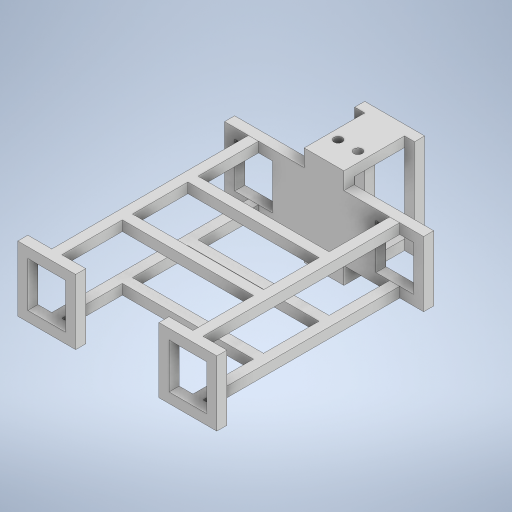
# Autodesk Inventor part: MTail
Saved by Autodesk Inventor 2024 (Build 280153000, 153)
## iProperties
Created: 2023-06-14
Part Number: MTail
Material: Generic
Document SubType Name: Modeling
Designer: vilas
Density: 1 g/cm^3
Appearance: Default
Author: vilas
Autodesk Inventor part; units mm, degrees
sketch "Sketch1" plane through (0, 0, 0) normal (0, 0, 1) x (1, 0, 0)
  line L0 (-32.5, 11.15) -> (32.5, 11.15) construction
  line L1 (32.5, 11.15) -> (32.5, -11.15) construction
  line L2 (32.5, -11.15) -> (-32.5, -11.15) construction
  line L3 (-32.5, -11.15) -> (-32.5, 11.15) construction
  line L4 (-32.5, 11.15) -> (32.5, -11.15) construction
  line L5 (32.5, 11.15) -> (-32.5, -11.15) construction
  line L6 (-32.5, 11.15) -> (-37.5, 11.15)
  line L7 (-37.5, 11.15) -> (-37.5, 16.15)
  line L8 (-37.5, 16.15) -> (-32.5, 16.15)
  line L9 (-32.5, 16.15) -> (-32.5, 11.15)
  line L10 (32.5, 11.15) -> (37.5, 11.15)
  line L11 (37.5, 11.15) -> (37.5, 16.15)
  line L12 (37.5, 16.15) -> (32.5, 16.15)
  line L13 (32.5, 16.15) -> (32.5, 11.15)
  line L14 (32.5, -11.15) -> (37.5, -11.15)
  line L15 (37.5, -11.15) -> (37.5, -16.15)
  line L16 (37.5, -16.15) -> (32.5, -16.15)
  line L17 (32.5, -16.15) -> (32.5, -11.15)
  line L18 (-32.5, -11.15) -> (-37.5, -11.15)
  line L19 (-37.5, -11.15) -> (-37.5, -16.15)
  line L20 (-37.5, -16.15) -> (-32.5, -16.15)
  line L21 (-32.5, -16.15) -> (-32.5, -11.15)
  point P0 (0, 0)
  dimension "d0" = 65
  dimension "d1" = 22.3
  dimension "d2" = 5
  dimension "d3" = 5
  dimension "d4" = 5
  dimension "d5" = 5
  dimension "d6" = 5
  dimension "d7" = 5
  dimension "d8" = 5
  dimension "d9" = 5
  constraints: 44 end point, 10 parallel, 5 horizontal, 5 perpendicular, 2 midpoint
  measures "d0" distance of L1.end L2.end
  measures "d1" distance of L0.end L1.end
  measures "d2" distance of L7.end L8.end
  measures "d3" distance of L6.end L7.end
  measures "d4" distance of L12.end L11.end
  measures "d5" distance of L11.end L10.end
  measures "d6" distance of L15.end L16.end
  measures "d7" distance of L14.end L15.end
  measures "d8" distance of L20.end L19.end
  measures "d9" distance of L19.end L18.end
extrude "Extrusion1" add sketch "Sketch1" along normal mid plane 97.524
ref_plane "Work Plane1" through (0, 0, 48.762) normal (0, 0, 1) x (1, 0, 0)
sketch "Sketch2" plane through (0, 0, 48.762) normal (0, 0, 1) x (1, 0, 0)
  line L0 (0, 0) -> (-35, 0) construction
  line L1 (0, 0) -> (35, 0) construction
  line L2 (-49.35, 16.15) -> (-20.65, 16.15)
  line L3 (-20.65, 16.15) -> (-20.65, -16.15)
  line L4 (-20.65, -16.15) -> (-49.35, -16.15)
  line L5 (-49.35, -16.15) -> (-49.35, 16.15)
  line L6 (-49.35, 16.15) -> (-20.65, -16.15) construction
  line L7 (-20.65, 16.15) -> (-49.35, -16.15) construction
  line L8 (20.65, 16.15) -> (49.35, 16.15)
  line L9 (49.35, 16.15) -> (49.35, -16.15)
  line L10 (49.35, -16.15) -> (20.65, -16.15)
  line L11 (20.65, -16.15) -> (20.65, 16.15)
  line L12 (20.65, 16.15) -> (49.35, -16.15) construction
  line L13 (49.35, 16.15) -> (20.65, -16.15) construction
  line L14 (-25.65, 11.15) -> (-44.35, 11.15)
  line L15 (-44.35, 11.15) -> (-44.35, -11.15)
  line L16 (-44.35, -11.15) -> (-25.65, -11.15)
  line L17 (-25.65, -11.15) -> (-25.65, 11.15)
  line L18 (44.35, 11.15) -> (25.65, 11.15)
  line L19 (25.65, 11.15) -> (25.65, -11.15)
  line L20 (25.65, -11.15) -> (44.35, -11.15)
  line L21 (44.35, -11.15) -> (44.35, 11.15)
  dimension "d13" = 35
  dimension "d14" = 35
  dimension "d15" = 28.7
  dimension "d16" = 32.3
  dimension "d17" = 28.7
  dimension "d18" = 32.3
  dimension "d19" = 5
  dimension "d20" = 5
  constraints: 44 end point, 8 parallel, 4 horizontal, 4 midpoint, 4 perpendicular, 6 other
  measures "d13" distance of L0.start L0.end
  measures "d14" distance of L0.start L1.end
  measures "d15" distance of L3.end L4.end
  measures "d16" distance of L2.end L3.end
  measures "d17" distance of L9.end L10.end
  measures "d18" distance of L8.end L9.end
  measures "d19" distance between parallel lines of L2 L14
  measures "d20" distance between parallel lines of L8 L18
extrude "Extrusion2" add sketch "Sketch2" along normal blind 5
ref_plane "Work Plane2" through (0, 0, -48.771) normal (0, 0, 1) x (1, 0, 0)
sketch "Sketch3" plane through (0, 0, -48.771) normal (0, 0, 1) x (1, 0, 0)
  line L0 (49.35, 16.15) -> (-49.35, 16.15)
  line L1 (-49.35, 16.15) -> (-49.35, -16.15)
  line L2 (-49.35, -16.15) -> (49.35, -16.15)
  line L3 (49.35, -16.15) -> (49.35, 16.15)
  line L4 (49.35, 16.15) -> (-49.35, -16.15) construction
  line L5 (-49.35, 16.15) -> (49.35, -16.15) construction
  line L6 (0, 0) -> (35, 0) construction
  line L7 (0, 0) -> (-35, 0) construction
  line L8 (32.5, -11.15) -> (25.65, -11.15) projected
  line L9 (44.35, 11.15) -> (25.65, 11.15)
  line L10 (25.65, 11.15) -> (25.65, -11.15)
  line L11 (25.65, -11.15) -> (44.35, -11.15)
  line L12 (44.35, -11.15) -> (44.35, 11.15)
  line L13 (44.35, 11.15) -> (25.65, -11.15) construction
  line L14 (25.65, 11.15) -> (44.35, -11.15) construction
  line L15 (-44.35, -11.15) -> (-44.35, 11.15) projected
  line L16 (-25.65, -11.15) -> (-44.35, -11.15)
  line L17 (-44.35, -11.15) -> (-44.35, 11.15)
  line L18 (-44.35, 11.15) -> (-25.65, 11.15)
  line L19 (-25.65, 11.15) -> (-25.65, -11.15)
  line L20 (-25.65, -11.15) -> (-44.35, 11.15) construction
  line L21 (-44.35, -11.15) -> (-25.65, 11.15) construction
  line L22 (0, 0) -> (0, 24.603) construction
  line L23 (0, 24.603) -> (9.85, 24.603) construction
  line L24 (9.85, 24.603) -> (-9.85, 24.603)
  line L25 (-9.85, 24.603) -> (-9.85, 16.15)
  line L26 (-9.85, 16.15) -> (9.85, 16.15)
  line L27 (9.85, 16.15) -> (9.85, 24.603)
  line L28 (0, 0) -> (0, -24.603) construction
  line L29 (0, -24.603) -> (9.85, -24.603) construction
  line L30 (9.85, -24.603) -> (-9.85, -24.603)
  line L31 (-9.85, -24.603) -> (-9.85, -16.15)
  line L32 (-9.85, -16.15) -> (9.85, -16.15)
  line L33 (9.85, -16.15) -> (9.85, -24.603)
  point P0 (30, -11.15)
  dimension "d24" = 98.7
  dimension "d25" = 32.3
  dimension "d26" = 35
  dimension "d27" = 35
  dimension "d76" = 24.603
  dimension "d77" = 9.85
  dimension "d78" = 19.7
  dimension "d79" = 24.603
  dimension "d80" = 9.85
  dimension "d81" = 19.7
  constraints: 64 end point, 10 parallel, 7 horizontal, 7 perpendicular, 6 midpoint, 3 point on line, 1 vertical
  measures "d24" distance of L2.end L1.end
  measures "d25" distance of L1.end L0.end
  measures "d26" distance of L6.start L6.end
  measures "d27" distance of L6.start L7.end
  measures "d76" distance of L6.start L22.end
  measures "d77" distance of L22.end L23.end
  measures "d78" distance of L26.end L25.end
  measures "d79" distance of L6.start L28.end
  measures "d80" distance of L28.end L29.end
  measures "d81" distance of L31.end L32.end
extrude "Extrusion3" add sketch "Sketch3" against normal blind 5
sketch "Sketch4" plane through (0, 0, 0) normal (1, 0, 0) x (0, 1, 0)
  line L0 (11.15, -48.762) -> (11.15, 48.762) projected
  line L1 (11.15, 18.754) -> (16.15, 18.754)
  line L2 (16.15, 18.754) -> (16.15, 13.754)
  line L3 (16.15, 13.754) -> (11.15, 13.754)
  line L4 (11.15, 13.754) -> (11.15, 18.754)
  line L5 (-16.15, 48.762) -> (16.15, 48.762) projected
  line L6 (11.15, -13.754) -> (16.15, -13.754)
  line L7 (16.15, -13.754) -> (16.15, -18.754)
  line L8 (16.15, -18.754) -> (11.15, -18.754)
  line L9 (11.15, -18.754) -> (11.15, -13.754)
  line L10 (16.15, -48.762) -> (11.15, -48.762) projected
  line L11 (-11.15, 48.762) -> (-11.15, -48.762) projected
  line L12 (-11.15, 18.754) -> (-16.15, 18.754)
  line L13 (-16.15, 18.754) -> (-16.15, 13.754)
  line L14 (-16.15, 13.754) -> (-11.15, 13.754)
  line L15 (-11.15, 13.754) -> (-11.15, 18.754)
  line L16 (-11.15, -18.754) -> (-16.15, -18.754)
  line L17 (-16.15, -18.754) -> (-16.15, -13.754)
  line L18 (-16.15, -13.754) -> (-11.15, -13.754)
  line L19 (-11.15, -13.754) -> (-11.15, -18.754)
  line L20 (-11.15, -48.762) -> (-16.15, -48.762) projected
  point P0 (0, 0)
  dimension "d30" = 5
  dimension "d31" = 5
  dimension "d32" = 30.008
  dimension "d33" = 5
  dimension "d34" = 5
  dimension "d35" = 30.008
  dimension "d36" = 5
  dimension "d37" = 5
  dimension "d38" = 5
  dimension "d39" = 5
  dimension "d40" = 30.008
  dimension "d41" = 30.008
  constraints: 32 end point, 8 parallel, 4 horizontal, 4 perpendicular, 4 point on line
  measures "d30" distance of L2.end L3.end
  measures "d31" distance of L1.end L2.end
  measures "d32" distance between parallel lines of L1 L5
  measures "d33" distance of L7.end L8.end
  measures "d34" distance of L6.end L7.end
  measures "d35" distance between parallel lines of L8 L10
  measures "d36" distance of L14.end L13.end
  measures "d37" distance of L13.end L12.end
  measures "d38" distance of L17.end L18.end
  measures "d39" distance of L16.end L17.end
  measures "d40" distance between parallel lines of L16 L20
  measures "d41" distance between parallel lines of L12 L5
extrude "Extrusion4" add sketch "Sketch4" along normal mid plane 65
sketch "Sketch7" plane through (0, 0, -53.771) normal (0, 0, -1) x (-1, 0, 0)
  line L0 (-9.85, 24.603) -> (9.85, 24.603)
  line L1 (9.85, 24.603) -> (9.85, -24.603)
  line L2 (9.85, -24.603) -> (-9.85, -24.603)
  line L3 (-9.85, -24.603) -> (-9.85, 24.603)
  line L4 (-9.85, 24.603) -> (9.85, -24.603) construction
  line L5 (9.85, 24.603) -> (-9.85, -24.603) construction
  line L6 (-9.85, 19.603) -> (9.85, 19.603)
  line L7 (-9.85, -19.603) -> (9.85, -19.603)
  point P0 (0, 0)
  point P1 (4.85, 24.603)
  point P2 (4.85, -24.603)
  point P3 (-4.85, 24.603)
  point P4 (-4.85, -24.603)
  dimension "d54" = 19.7
  dimension "d55" = 49.206
  dimension "d74" = 5
  dimension "d75" = 5
  constraints: 16 end point, 8 point on line, 3 perpendicular, 2 midpoint, 2 parallel, 1 horizontal
  measures "d54" distance of L1.end L2.end
  measures "d55" distance of L0.end L1.end
  measures "d74" distance between parallel lines of L6 L0
  measures "d75" distance between parallel lines of L2 L7
extrude "Extrusion7" add sketch "Sketch7" along normal blind 25 contours L0 L1 L6 L3 | L7 L1 L2 L3
ref_plane "Work Plane3" through (0, 0, -78.771) normal (0, 0, -1) x (-1, 0, 0)
sketch "Sketch8" plane through (0, 0, -78.771) normal (0, 0, -1) x (-1, 0, 0)
  line L0 (-14.85, 24.603) -> (14.85, 24.603)
  line L1 (14.85, 24.603) -> (14.85, -24.603)
  line L2 (14.85, -24.603) -> (-14.85, -24.603)
  line L3 (-14.85, -24.603) -> (-14.85, 24.603)
  line L4 (-14.85, 24.603) -> (14.85, -24.603) construction
  line L5 (14.85, 24.603) -> (-14.85, -24.603) construction
  line L6 (9.85, 19.603) -> (-9.85, 19.603)
  line L7 (-9.85, 19.603) -> (-9.85, -19.603)
  line L8 (-9.85, -19.603) -> (9.85, -19.603)
  line L9 (9.85, -19.603) -> (9.85, 19.603)
  point P0 (0, 0)
  dimension "d61" = 29.7
  dimension "d62" = 49.206
  dimension "d63" = 5
  constraints: 20 end point, 4 parallel, 2 midpoint, 2 perpendicular, 1 horizontal, 3 other
  measures "d61" distance of L1.end L2.end
  measures "d62" distance of L0.end L1.end
  measures "d63" distance between parallel lines of L0 L6
extrude "Extrusion8" add sketch "Sketch8" along normal blind 5
sketch "Sketch10" plane through (0, 0, 0) normal (0, 1, 0) x (-1, 0, 0)
  circle A0 centre (-4.925, -60.66) radius 2.1
  line L0 (-9.85, -53.771) -> (9.85, -53.771) projected
  line L1 (-9.85, -53.771) -> (-9.85, -78.771) projected
  circle A1 centre (4.925, -60.66) radius 2.1
  line L2 (9.85, -53.771) -> (9.85, -78.771) projected
  point P0 (0, 0)
  dimension "d82" = 4.2
  dimension "d83" = 6.889
  dimension "d84" = 4.925
  dimension "d85" = 4.2
  dimension "d86" = 6.889
  dimension "d87" = 4.925
  constraints: 2 centre point
  measures "d82" diameter of A0
  measures "d83" distance from line of L0 A0.centre
  measures "d84" distance from line of A0.centre L1
  measures "d85" diameter of A1
  measures "d86" distance from line of L0 A1.centre
  measures "d87" distance from line of A1.centre L2
extrude "Extrusion10" cut sketch "Sketch10" along normal through all both and the other way through all
body "Solid1"
